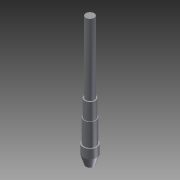
# Autodesk Inventor part: Collect_Jaw
Saved by Autodesk Inventor 2011 SP2 (Build 150309200, 309)
## iProperties
Created: 2012-02-15
Part Number: Collect_Jaw
Document SubType Name: Modeling
Designer: sungwook
Density: 1 g/cm^3
Author: sungwook
Autodesk Inventor part; units mm, degrees
ref_plane "YZ Plane" through (0, 0, 0) normal (1, 0, 0) x (0, 1, 0)
ref_plane "XZ Plane" through (0, 0, 0) normal (0, 1, 0) x (-1, 0, 0)
ref_plane "XY Plane" through (0, 0, 0) normal (0, 0, 1) x (1, 0, 0)
sketch "Sketch1" plane through (0, 0, 0) normal (0, 0, 1) x (1, 0, 0)
  circle A0 centre (0, 0) radius 4.125
  dimension "d0" = 8.25
  constraints: 1 centre point, 1 coincident
  measures "d0" diameter of A0
extrude "Extrusion1" add sketch "Sketch1" along normal blind 77
sketch "Sketch2" plane through (0, 0, 0) normal (1, 0, 0) x (0, 1, 0)
  line L0 (-4.125, 0) -> (-4.125, 77) projected
  line L1 (4.125, 0) -> (4.125, 77) projected
  line L2 (0, -15.4) -> (0, 92.4) projected
  line L3 (-5.775, 0) -> (5.775, 0) projected
  line L4 (2.4, 0) -> (0, 0)
  line L5 (0, 5.6) -> (4.125, 5.6)
  line L6 (4.125, 5.6) -> (4.125, 0)
  line L7 (-4.125, 0) -> (-4.125, 5.6)
  line L8 (-4.125, 5.6) -> (-2.4, 0)
  line L9 (4.125, 0) -> (0, 0)
  line L10 (-2.4, 0) -> (-4.125, 0)
  point P0 (0, 3.0897)
  dimension "d4" = 5.6
  constraints: 14 end point, 5 point on line, 3 parallel, 1 horizontal, 1 perpendicular, 1 vertical alignment
  measures "d4" distance of L1.start L5.end
revolve "Revolution1" cut sketch "Sketch2" angle 360 about axis through (0, 0, -10) along (0, 0, 1) contours L0 L8 L3
sketch "Sketch3" plane through (0, 0, 77) normal (0, 0, 1) x (1, 0, 0)
  circle A0 centre (0, 0) radius 4.125 projected
  circle A1 centre (0, 0) radius 2.5
  dimension "d19" = 5
  constraints: 1 centre point, 1 coincident
  measures "d19" diameter of A1
extrude "Extrusion2" cut sketch "Sketch3" against normal blind 42.5
sketch "Sketch4" plane through (0, 0, 34.5) normal (0, 0, 1) x (1, 0, 0)
  circle A0 centre (0, 0) radius 4.125 projected
  circle A1 centre (0, 0) radius 3.135
  dimension "d22" = 6.27
  constraints: 1 centre point, 1 coincident
  measures "d22" diameter of A1
extrude "Extrusion3" cut sketch "Sketch4" against normal blind 10
sketch "Sketch5" plane through (0, 0, 24.5) normal (0, 0, 1) x (1, 0, 0)
  circle A0 centre (0, 0) radius 4.125 projected
  circle A1 centre (0, 0) radius 3.5
  dimension "d25" = 7
  constraints: 1 centre point, 1 coincident
  measures "d25" diameter of A1
extrude "Extrusion4" cut sketch "Sketch5" against normal blind 13.5
body "Solid1"
